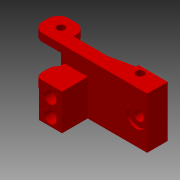
# Autodesk Inventor part: exTop
Saved by Autodesk Inventor 2013 (Build 170138000, 138)
## iProperties
Created: 2015-01-15
Part Number: exTop
Material: Generic
Document SubType Name: Modeling
Designer: dzban
Density: 1 g/cm^3
Author: dzban
Autodesk Inventor part; units mm, degrees
ref_plane "YZ Plane" through (0, 0, 0) normal (1, 0, 0) x (0, 1, 0)
ref_plane "XZ Plane" through (0, 0, 0) normal (0, 1, 0) x (-1, 0, 0)
ref_plane "XY Plane" through (0, 0, 0) normal (0, 0, 1) x (1, 0, 0)
sketch "Sketch1" plane through (0, 0, 0) normal (0, 0, 1) x (1, 0, 0)
  line L0 (-17.1448, -21) -> (23.7, -21)
  line L1 (23.7, -21) -> (23.7, -13)
  line L2 (23.7, -13) -> (12.3117, -13)
  line L3 (12.3117, -13) -> (12.3117, -14)
  line L4 (12.3117, -14) -> (3.1793, -16)
  line L5 (3.1793, -16) -> (-10.1347, -16)
  line L6 (-10.1347, -16) -> (-10.1347, -14.8234)
  arc A0 (-10.1347, -14.8234) -> (-14.1347, -10.8234) centre (-14.1347, -14.8234) ccw
  line L7 (-14.1347, -10.8234) -> (-17.1448, -10.8234)
  arc A1 (-17.1448, -10.8234) -> (-21.1448, -14.8234) centre (-17.1448, -14.8234) ccw
  line L8 (-21.1448, -14.8234) -> (-21.1448, -17)
  arc A2 (-21.1448, -17) -> (-17.1448, -21) centre (-17.1448, -17) ccw
  circle A3 centre (-15.5, -15.5) radius 1.5
  circle A4 centre (15.3552, -15.5) radius 1.5
  point P0 (0, 0)
  constraints: 18 end point, 6 point on circle, 5 centre point
extrude "Extrusion1" add sketch "Sketch1" along normal blind 3
sketch "Sketch2" plane through (0, 0, 3) normal (0, 0, 1) x (1, 0, 0)
  circle A0 centre (15.3552, -15.5) radius 1.5 projected
  line L0 (-10, -16) -> (-10, -21)
  line L1 (23.7, -21) -> (-10, -21)
  line L2 (23.7, -13) -> (23.7, -21)
  line L3 (12.3117, -13) -> (23.7, -13)
  line L4 (12.3117, -14) -> (12.3117, -13)
  line L5 (3.1793, -16) -> (12.3117, -14)
  line L6 (-10, -16) -> (3.1793, -16)
  circle A1 centre (15.5, -15.5) radius 1.5
  point P0 (0, 0)
  constraints: 14 end point, 1 centre point
extrude "Extrusion2" add sketch "Sketch2" along normal blind 14
sketch "Sketch4" plane through (0, 0, 17) normal (0, 0, 1) x (1, 0, 0)
  line L0 (-10, -16) -> (-10, -21) projected
  line L1 (-10, -21) -> (23.7, -21) projected
  line L2 (23.7, -21) -> (23.7, -13) projected
  line L3 (23.7, -13) -> (12.3117, -13) projected
  line L4 (12.3117, -13) -> (12.3117, -14) projected
  line L5 (12.3117, -14) -> (3.1793, -16) projected
  line L6 (3.1793, -16) -> (-10, -16) projected
  arc A0 (15.4276, -14.0017) -> (15.4276, -16.9983) centre (15.3552, -15.5) ccw projected
  arc A1 (15.4276, -16.9983) -> (15.4276, -14.0017) centre (15.5, -15.5) ccw projected
  line L7 (-10, -21) -> (-10, -16) projected
  line L8 (-10, -16) -> (-10.1347, -16) projected
  line L9 (-10.1347, -16) -> (-10.1347, -14.8234) projected
  arc A2 (-10.1347, -14.8234) -> (-14.1347, -10.8234) centre (-14.1347, -14.8234) ccw projected
  line L10 (-14.1347, -10.8234) -> (-17.1448, -10.8234) projected
  arc A3 (-17.1448, -10.8234) -> (-21.1448, -14.8234) centre (-17.1448, -14.8234) ccw projected
  line L11 (-21.1448, -14.8234) -> (-21.1448, -17) projected
  arc A4 (-21.1448, -17) -> (-17.1448, -21) centre (-17.1448, -17) ccw projected
  line L12 (-17.1448, -21) -> (-10, -21) projected
  circle A5 centre (-15.5, -15.5) radius 1.5 projected
  point P0 (0, 0)
extrude "Extrusion3" add sketch "Sketch4" along normal blind 3
sketch "Sketch5" plane through (-17.1448, -21, 0) normal (0, -1, 0) x (1, 0, 0)
  line L0 (7.1448, 3) -> (7.1448, 17) projected
  circle A0 centre (12.889, 3.3484) radius 2.5
  circle A1 centre (12.889, 9.9795) radius 2.5
  line L1 (8.5448, -0.0205) -> (17.5875, -0.0205)
  line L2 (17.5875, -0.0205) -> (17.5875, 14.0778)
  line L3 (17.5875, 14.0778) -> (8.5448, 14.0778)
  line L4 (8.5448, 14.0778) -> (8.5448, -0.0205)
  point P0 (17.1448, 0)
  point P1 (17.1448, -14)
  dimension "d6" = 5
  dimension "d8" = 5
  dimension "d9" = 4.0983
  dimension "d10" = 4.6985
  dimension "d11" = 3.3689
  dimension "d12" = 4.3442
  dimension "d13" = 6.6311
  dimension "d14" = 1.4
  constraints: 8 end point, 2 centre point, 2 horizontal, 2 vertical, 1 vertical alignment
  measures "d6" diameter of A1
  measures "d8" diameter of A0
  measures "d9" distance from line of L3 A1.centre
  measures "d10" distance from line of L2 A1.centre
  measures "d11" distance from line of L1 A0.centre
  measures "d12" distance from line of L4 A0.centre
  measures "d13" distance of A1.centre A0.centre
  measures "d14" distance between parallel lines of L4 L0
extrude "Extrusion4" add sketch "Sketch5" along normal blind 10
sketch "Sketch6" plane through (-4.2558, -21, 9.9795) normal (0, -1, 0) x (1, 0, 0)
  circle A0 centre (0, 0) radius 2.5 projected
  circle A1 centre (0, 0) radius 1
  point P0 (4.2558, -9.9795)
  dimension "d17" = 2
  constraints: 1 centre point, 1 coincident
  measures "d17" diameter of A1
extrude "Extrusion5" cut sketch "Sketch6" against normal blind 10 contours A1
sketch "Sketch7" plane through (-17.1448, -21, 0) normal (0, -1, 0) x (1, 0, 0)
  line L0 (17.5875, 0) -> (40.8448, 0) projected
  line L1 (40.8448, 0) -> (40.8448, 20) projected
  circle A0 centre (36.5448, 10) radius 4
  point P0 (17.1448, 0)
  dimension "d21" = 4.3
  dimension "d22" = 10
  dimension "d23" = 8
  constraints: 1 centre point
  measures "d21" distance from line of L1 A0.centre
  measures "d22" distance from line of A0.centre L0
  measures "d23" diameter of A0
extrude "Extrusion6" cut sketch "Sketch7" against normal blind 1
sketch "Sketch8" plane through (19.4, -20, 10) normal (0, -1, 0) x (1, 0, 0)
  circle A0 centre (0, 0) radius 4 projected
  circle A1 centre (0, 0) radius 2
  point P0 (-19.4, -10)
  dimension "d26" = 4
  constraints: 1 centre point, 1 coincident
  measures "d26" diameter of A1
extrude "Extrusion7" cut sketch "Sketch8" against normal blind 11 contours A1
body "Solid1"
